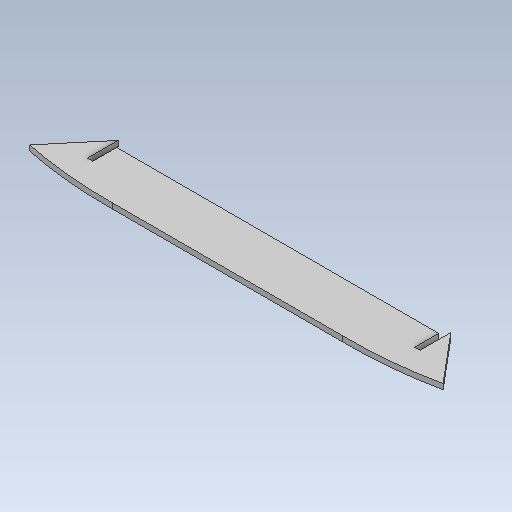
# Autodesk Inventor part: transom
Saved by Autodesk Inventor 2020.3 (Build 243373000, 373)
## iProperties
Created: 2020-05-22
Part Number: transom
Material: Generic
Document SubType Name: Modeling
Designer: kardo
Density: 1 g/cm^3
Appearance: Default
Mass: 5.21087 g
Surface Area: 59.464 cm^2
Volume: 5.21087 cm^3
Author: kardo
Autodesk Inventor part; units mm, degrees
ref_plane "YZ Plane" through (0, 0, 0) normal (1, 0, 0) x (0, 1, 0)
ref_plane "XZ Plane" through (0, 0, 0) normal (0, 1, 0) x (-1, 0, 0)
ref_plane "XY Plane" through (0, 0, 0) normal (0, 0, 1) x (1, 0, 0)
derived "base_sketch.ipt"
sketch "transom" plane through (0, -306, 31.875) normal (0, 1, 0) x (-1, 0, 0)
  line L0 (19.176, 14.943) -> (62.322, 14.943)
  line L1 (62.322, 14.943) -> (62.322, -18.346)
  line L2 (28.764, -18.346) -> (62.322, -18.346)
  line L3 (0, -20.4) -> (-15.1069, -2.3963)
  line L4 (0, -20.4) -> (0, -17.85)
  line L5 (0, -17.85) -> (62.322, -17.85)
  line L6 (62.322, 0.918) -> (19.176, 0.918)
  line L7 (19.176, 14.943) -> (19.176, 0.918) construction
  line L8 (-19.176, -3.3048) -> (-19.176, 10.7202) construction
  line L9 (-38.352, 4.845) -> (-38.352, -9.18) construction
  line L10 (0, 14.025) -> (0, 0) construction
  spline S0 degree 4 poles (-57.528, -4.335) (-46.0483, 2.3301) (-30.6129, 8.6531) (-11.2214, 13.1664) (8.3201, 14.943) (15.5662, 14.943) (19.176, 14.943) knots 0 0 0 0 0 0.630279 0.815816 1 1 1 1 1
  spline S1 degree 3 poles (19.176, 0.918) (-0.1981, 1.1561) (-19.6083, -2.0969) (-38.352, -9.18) knots 0 0 0 0 1 1 1 1
  point P0 (0, -31.875)
ref_plane "transom_plane" through (0, -306, 31.875) normal (0, 1, 0) x (-1, 0, 0)
sketch "Sketch2" plane through (0, -306, 31.875) normal (0, 1, 0) x (-1, 0, 0)
  line L0 (0, -20.4) -> (-15.1069, -2.3963) projected
  line L1 (0, -17.85) -> (62.322, -17.85) projected
  line L2 (0, -20.4) -> (0, -17.85) projected
  spline S0 degree 3 poles (19.176, 0.918) (-0.1981, 1.1561) (-19.6083, -2.0969) (-38.352, -9.18) knots 0 0 0 0 1 1 1 1 projected
  line L3 (62.322, 0.918) -> (19.176, 0.918) projected
  line L4 (62.322, 14.943) -> (62.322, -18.346) projected
  line L5 (0, -17.85) -> (0, -8.925)
  line L6 (0, -8.925) -> (2, -8.925)
  line L7 (2, -8.925) -> (2, -17.85)
  line L8 (0, -8.925) -> (0, 0) construction
  point P0 (0, -31.875)
  dimension "d1" = 2
  constraints: 8 end point, 3 collinear, 2 parallel, 1 point on line, 1 other
  measures "d1" distance of L5.end L6.end
extrude "Extrusion1" add sketch "Sketch2" along normal blind 2 contours L0 S0 L3 L4 L1 L7 L6 L5 L2
mirror "Mirror1" about plane through (-62.322, -306, 14.025) normal (-1, 0, 0) of "Extrusion1"
equation "\"d1\" = stringer_thickness"
equation "\"d2\" = bulkhead_thickness"
equation "\"stringer_thickness\" = 2"
equation "\"bulkhead_thickness\" = 2"
body "Solid1"
